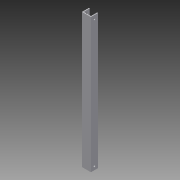
# Autodesk Inventor part: Rack - Back
Saved by Autodesk Inventor 2013 (Build 170138000, 138)
## iProperties
Created: 2013-01-08
Part Number: Rack - Back
Material: Generic
Document SubType Name: Modeling
Designer: Naphat
Density: 1 g/cm^3
Author: Naphat
Autodesk Inventor part; units mm, degrees
ref_plane "YZ Plane" through (0, 0, 0) normal (1, 0, 0) x (0, 1, 0)
ref_plane "XZ Plane" through (0, 0, 0) normal (0, 1, 0) x (-1, 0, 0)
ref_plane "XY Plane" through (0, 0, 0) normal (0, 0, 1) x (1, 0, 0)
sketch "Sketch1" plane through (0, 0, 0) normal (0, 0, 1) x (1, 0, 0)
  line L0 (-16, 12.5) -> (-13, 12.5)
  line L1 (-13, 12.5) -> (-13, -9.5)
  line L2 (-13, -9.5) -> (13, -9.5)
  line L3 (13, -9.5) -> (13, 12.9)
  line L4 (13, 12.9) -> (16, 12.9)
  line L5 (16, 12.9) -> (16, -12.5)
  line L6 (16, -12.5) -> (-16, -12.5)
  line L7 (-16, -12.5) -> (-16, 12.5)
  point P0 (0, 0)
  dimension "d0" = 3
  dimension "d2" = 3
  dimension "d3" = 25
  dimension "d4" = 32
  dimension "d5" = 16
  dimension "d7" = 12.5
  dimension "d8" = 3
  constraints: 16 end point, 6 parallel, 1 horizontal, 1 perpendicular
  measures "d0" distance of L0.start L0.end
  measures "d2" distance of L3.end L4.end
  measures "d3" distance of L6.end L0.start
  measures "d4" distance of L5.end L6.end
  measures "d5" distance from line of point (0, 0) L7
  measures "d7" distance from line of L6 point (0, 0)
  measures "d8" distance between parallel lines of L6 L2
extrude "Extrusion1" add sketch "Sketch1" against normal blind 482.6
sketch "Sketch4" plane through (16, -12.5, 0) normal (1, 0, 0) x (0, 0, -1)
  line L0 (0, 25.4) -> (0, 0) projected
  line L1 (482.6, 25.4) -> (482.6, 0) projected
  line L2 (0, 25.4) -> (482.6, 25.4) projected
  circle A0 centre (12.7, 12.7) radius 3.175
  circle A1 centre (469.9, 12.7) radius 3.175
  point P0 (0, 12.5)
  dimension "d21" = 6.35
  dimension "d24" = 12.7
  dimension "d26" = 12.7
  dimension "d27" = 6.35
  dimension "d28" = 12.7
  dimension "d29" = 12.7
  constraints: 2 centre point
  measures "d21" diameter of A0
  measures "d24" distance from line of A1.centre L2
  measures "d26" distance from line of A0.centre L2
  measures "d27" diameter of A1
  measures "d28" distance from line of L0 A0.centre
  measures "d29" distance from line of L1 A1.centre
hole "Mount Hole" at (16, 0.2, -12.7) at (16, 0.2, -469.9) direction (-1, 0, 0) diameter 6.35 depth 12.7 tip angle 118
sketch "Sketch5" plane through (-16, -12.5, 0) normal (-1, 0, 0) x (0, 0, 1)
  circle A0 centre (-12.7, 12.7) radius 3.175 projected
  circle A1 centre (-469.9, 12.7) radius 3.175 projected
  circle A2 centre (-469.9, 12.7) radius 4.7625
  circle A3 centre (-12.7, 12.7) radius 4.7625
  point P0 (0, 12.5)
  dimension "d37" = 9.525
  dimension "d38" = 9.525
  constraints: 2 centre point, 2 coincident
  measures "d37" diameter of A2
  measures "d38" diameter of A3
hole "Access Hole" at (-16, 0.2, -469.9) at (-16, 0.2, -12.7) direction (1, 0, 0) diameter 9.525 depth 3 tip angle 118
sketch "Sketch6" plane through (-16, -12.5, 0) normal (-1, 0, 0) x (0, 0, 1)
  line L0 (0, 0) -> (0, 25) projected
  line L1 (-482.6, 0) -> (-482.6, 25) projected
  line L2 (0, 0) -> (-482.6, 0) projected
  circle A0 centre (-431.519, 15.5) radius 3.175
  circle A1 centre (-51.081, 15.5) radius 3.175
  point P0 (0, 12.5)
  dimension "d46" = 6.35
  dimension "d47" = 51.081
  dimension "d48" = 15.5
  dimension "d49" = 6.35
  dimension "d50" = 51.081
  constraints: 2 centre point, 1 horizontal alignment
  measures "d46" diameter of A0
  measures "d47" distance from line of L1 A0.centre
  measures "d48" distance from line of A0.centre L2
  measures "d49" diameter of A1
  measures "d50" distance from line of L0 A1.centre
hole "Hole3" at (-16, 3, -431.519) at (-16, 3, -51.081) direction (1, 0, 0) diameter 6.35 depth 3 tip angle 118
equation "\"d2\" = d0"
equation "\"d5\" = 0.5 * d4"
equation "\"d7\" = 0.5 * d3"
equation "\"d8\" = d0"
equation "\"d24\" = d26"
equation "\"d27\" = d21"
equation "\"d28\" = d26"
equation "\"d29\" = d24"
equation "\"d35\" = d24"
equation "\"d38\" = d37"
equation "\"d50\" = d47"
body "Solid1"
